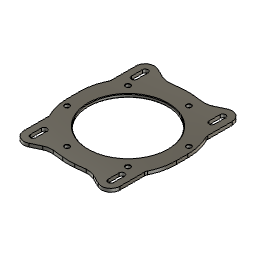
Motor_Base_Plate_Botm v4 (Autodesk Fusion 360 design; units mm, degrees)
Autodesk Fusion 360 part; units mm, degrees
sketch "Sketch1" plane through (0, 0, 0) normal (0, 0, 1) x (1, 0, 0)
  line L0 (0, 0) -> (42.0984, 0) construction
  line L1 (0, 2.5) -> (0, 20)
  line L2 (20, 0) -> (2.5, 0)
  line L3 (43.5453, 45.7571) -> (43.5453, 28.6506)
  arc A0 (32.6927, 46.2539) -> (32.6429, 45.7571) centre (35.1429, 45.7571) ccw
  arc A1 (-32.6429, 45.7571) -> (-32.7077, 46.3226) centre (-35.1429, 45.7571) ccw
  line L4 (-43.5453, 45.7571) -> (-43.5453, 28.6506)
  line L5 (16.6515, 53.2283) -> (16.6515, 59.0493) construction
  line L6 (-15.557, 53.706) -> (-15.557, 59.527) construction
  line L7 (0, 0) -> (45, 0) construction
  arc A2 (-41.8537, 25.4807) -> (-42.1265, 25.0272) centre (0, 0) ccw
  arc A3 (4.0267, 61.4469) -> (-4.7848, 61.3754) centre (-0.036, 19.1415) ccw
  arc A4 (43.4103, 49.257) -> (33.6006, 59.0168) centre (35.1429, 50.7571) ccw
  line L8 (16.6515, 58.2283) -> (16.6515, 64.0493) construction
  arc A5 (28.1023, 59.5419) -> (33.6006, 59.0168) centre (31.7651, 68.8469) ccw
  arc A6 (14.9315, 52.7652) -> (22.9245, 54.1858) centre (16.401, 67.693) ccw
  line L9 (-22.9245, 54.1858) -> (-31.3596, 58.2597)
  arc A7 (49, 5) -> (41.8537, 30.4807) centre (0, 5) ccw
  line L10 (43.5453, 50.7571) -> (43.5453, 28.6506)
  line L11 (14.9315, 52.7652) -> (5.4274, 53.7007)
  line L12 (-41.2861, 38.5638) -> (-43.4103, 49.257)
  arc A8 (-9.7818, 62.096) -> (-4.7848, 61.3754) centre (-5.9022, 71.3127) ccw
  line L13 (-14.9315, 52.7652) -> (-5.4274, 53.7007)
  arc A9 (-37.6429, 40.7571) -> (-32.6429, 40.7571) centre (-35.1429, 40.7571) ccw
  circle A10 centre (-15.557, 58.706) radius 1.5
  line L14 (-43.5453, 50.7571) -> (-43.5453, 28.6506)
  arc A11 (-44.0504, 26.4608) -> (-43.5453, 28.6506) centre (-48.5453, 28.6506) ccw
  arc A12 (-32.6429, 50.7571) -> (-37.6429, 50.7571) centre (-35.1429, 50.7571) ccw
  line L15 (-19.3563, 63.0202) -> (-28.095, 59.5544)
  arc A13 (-33.6082, 59.0182) -> (-28.095, 59.5544) centre (-31.7817, 68.85) ccw
  line L16 (-7.2407, 61.0264) -> (-0.4717, 58.2301) construction
  arc A14 (-11.79, 62.9413) -> (-19.3563, 63.0202) centre (-15.6696, 53.7246) ccw
  arc A15 (43.5453, 28.6506) -> (44.0504, 26.4608) centre (48.5453, 28.6506) ccw
  line L17 (-11.79, 62.9413) -> (-9.7818, 62.096)
  line L18 (41.2861, 38.5638) -> (43.4103, 49.257)
  arc A16 (-7.2407, 61.0264) -> (6.4194, 61.1484) centre (-0.036, 19.1415) ccw construction
  arc A17 (-22.9245, 54.1858) -> (-14.9315, 52.7652) centre (-16.401, 67.693) ccw
  arc A18 (41.2861, 38.5638) -> (41.8537, 30.4807) centre (56.0268, 35.5374) ccw
  line L19 (-15.557, 58.706) -> (-15.557, 64.527) construction
  line L20 (11.1293, 63.1457) -> (8.8867, 62.1947)
  arc A19 (4.0267, 61.4469) -> (8.8867, 62.1947) centre (4.9826, 71.4011) ccw
  line L21 (6.4194, 61.1484) -> (-0.4717, 58.2301) construction
  arc A20 (43.4103, 49.257) -> (31.3596, 58.2597) centre (35.1429, 50.7571) ccw
  line L22 (-37.6429, 50.7571) -> (-37.6429, 40.7571)
  arc A21 (-33.6006, 59.0168) -> (-43.4103, 49.257) centre (-35.1429, 50.7571) ccw
  arc A22 (-41.8537, 30.4807) -> (-41.2861, 38.5638) centre (-56.0268, 35.5374) ccw
  arc A23 (-31.3596, 58.2597) -> (-43.4103, 49.257) centre (-35.1429, 50.7571) ccw
  arc A24 (18.6963, 63.2444) -> (11.1293, 63.1457) centre (15.0335, 53.9393) ccw
  arc A25 (5.4274, 53.7007) -> (-5.4274, 53.7007) centre (0, 5) ccw
  circle A26 centre (16.6515, 58.2283) radius 1.5
  arc A27 (-41.8537, 30.4807) -> (-49, 5) centre (0, 5) ccw
  line L23 (18.6963, 63.2444) -> (28.1023, 59.5419)
  line L24 (22.9245, 54.1858) -> (31.3596, 58.2597)
  arc A28 (-33.6006, 54.0168) -> (-33.6082, 54.0182) centre (-35.1429, 45.7571) ccw
  line L25 (32.6429, 45.7571) -> (32.6429, 40.7571)
  line L26 (32.6429, 50.7571) -> (32.6429, 45.7571)
  line L27 (37.6429, 50.7571) -> (37.6429, 40.7571)
  arc A29 (37.6429, 50.7571) -> (32.6429, 50.7571) centre (35.1429, 50.7571) ccw
  arc A30 (32.6429, 40.7571) -> (37.6429, 40.7571) centre (35.1429, 40.7571) ccw
  arc A31 (-5.4274, -53.7007) -> (5.4274, -53.7007) centre (0, -5) ccw
  arc A32 (22.9245, -54.1858) -> (14.9315, -52.7652) centre (16.401, -67.693) ccw
  line L28 (-15.557, -53.706) -> (-15.557, -59.527) construction
  arc A33 (31.3596, -58.2597) -> (43.4103, -49.257) centre (35.1429, -50.7571) ccw
  line L29 (6.4194, -61.1484) -> (-0.4717, -58.2301) construction
  circle A34 centre (16.6515, -58.2283) radius 1.5
  arc A35 (-49, -5) -> (-41.8537, -30.4807) centre (0, -5) ccw
  arc A36 (-42.1265, -25.0272) -> (-41.8537, -25.4807) centre (0, 0) ccw
  line L30 (-11.79, -62.9413) -> (-9.7818, -62.096)
  arc A37 (8.8867, -62.1947) -> (4.0267, -61.4469) centre (4.9826, -71.4011) ccw
  arc A38 (-41.2861, -38.5638) -> (-41.8537, -30.4807) centre (-56.0268, -35.5374) ccw
  line L31 (11.1293, -63.1457) -> (8.8867, -62.1947)
  arc A39 (-43.5453, -28.6506) -> (-44.0504, -26.4608) centre (-48.5453, -28.6506) ccw
  line L32 (-22.9245, -54.1858) -> (-31.3596, -58.2597)
  arc A40 (-19.3563, -63.0202) -> (-11.79, -62.9413) centre (-15.6696, -53.7246) ccw
  arc A41 (-33.6082, -54.0182) -> (-33.6006, -54.0168) centre (-35.1429, -45.7571) ccw
  arc A42 (-4.7848, -61.3754) -> (4.0267, -61.4469) centre (-0.036, -19.1415) ccw
  line L33 (22.9245, -54.1858) -> (31.3596, -58.2597)
  line L34 (-15.557, -58.706) -> (-15.557, -64.527) construction
  line L35 (-43.5453, -45.7571) -> (-43.5453, -28.6506)
  line L36 (14.9315, -52.7652) -> (5.4274, -53.7007)
  arc A43 (-14.9315, -52.7652) -> (-22.9245, -54.1858) centre (-16.401, -67.693) ccw
  line L37 (43.5453, -45.7571) -> (43.5453, -28.6506)
  line L38 (-43.5453, -50.7571) -> (-43.5453, -28.6506)
  arc A44 (-43.5453, -23.6506) -> (-44.0504, -21.4608) centre (-48.5453, -23.6506) ccw
  line L39 (41.2861, -38.5638) -> (43.4103, -49.257)
  arc A45 (-28.095, -59.5544) -> (-33.6082, -59.0182) centre (-31.7817, -68.85) ccw
  arc A46 (-4.7848, -61.3754) -> (-9.7818, -62.096) centre (-5.9022, -71.3127) ccw
  line L40 (20, 0) -> (2.5, 0)
  line L41 (16.6515, -53.2283) -> (16.6515, -59.0493) construction
  line L42 (18.6963, -63.2444) -> (28.1023, -59.5419)
  arc A47 (33.6006, -59.0168) -> (43.4103, -49.257) centre (35.1429, -50.7571) ccw
  line L43 (-7.2407, -61.0264) -> (-0.4717, -58.2301) construction
  arc A48 (41.8537, -30.4807) -> (49, -5) centre (0, -5) ccw
  arc A49 (-43.4103, -49.257) -> (-33.6006, -59.0168) centre (-35.1429, -50.7571) ccw
  line L44 (16.6515, -58.2283) -> (16.6515, -64.0493) construction
  arc A50 (44.0504, -26.4608) -> (43.5453, -28.6506) centre (48.5453, -28.6506) ccw
  circle A51 centre (-15.557, -58.706) radius 1.5
  line L45 (-41.2861, -38.5638) -> (-43.4103, -49.257)
  arc A52 (41.8537, -30.4807) -> (41.2861, -38.5638) centre (56.0268, -35.5374) ccw
  arc A53 (33.6006, -59.0168) -> (28.1023, -59.5419) centre (31.7651, -68.8469) ccw
  line L46 (-19.3563, -63.0202) -> (-28.095, -59.5544)
  arc A54 (6.4194, -61.1484) -> (-7.2407, -61.0264) centre (-0.036, -19.1415) ccw construction
  line L47 (-14.9315, -52.7652) -> (-5.4274, -53.7007)
  arc A55 (-43.4103, -49.257) -> (-31.3596, -58.2597) centre (-35.1429, -50.7571) ccw
  line L48 (43.5453, -50.7571) -> (43.5453, -28.6506)
  arc A56 (11.1293, -63.1457) -> (18.6963, -63.2444) centre (15.0335, -53.9393) ccw
  line L49 (49, 5) -> (49, -5)
  line L50 (-49, -5) -> (-49, 5)
  circle A57 centre (0, 0) radius 45
  line L51 (0, 0) -> (11.6469, 43.4667) construction
  line L52 (0, 0) -> (45, 0) construction
  circle A58 centre (11.6469, 43.4667) radius 2
  circle A59 centre (-31.8198, 31.8198) radius 2
  circle A60 centre (-43.4667, -11.6469) radius 2
  circle A61 centre (-11.6469, -43.4667) radius 2
  circle A62 centre (31.8198, -31.8198) radius 2
  circle A63 centre (43.4667, 11.6469) radius 2
  circle A64 centre (0, 0) radius 35.75
  line L53 (-35.1429, 45.7571) -> (-35.1429, 50.7571)
  line L54 (-35.1429, 45.7571) -> (-35.1429, 40.7571)
  line L55 (-32.6429, 50.7571) -> (-32.6429, 40.7571)
  line L56 (37.6429, -50.7571) -> (37.6429, -40.7571)
  arc A65 (32.6429, -50.7571) -> (37.6429, -50.7571) centre (35.1429, -50.7571) ccw
  line L57 (32.6429, -50.7571) -> (32.6429, -45.7571)
  line L58 (32.6429, -45.7571) -> (32.6429, -40.7571)
  arc A66 (37.6429, -40.7571) -> (32.6429, -40.7571) centre (35.1429, -40.7571) ccw
  line L59 (-32.6429, -50.7571) -> (-32.6429, -40.7571)
  line L60 (-37.6429, -50.7571) -> (-37.6429, -40.7571)
  arc A67 (-37.6429, -50.7571) -> (-32.6429, -50.7571) centre (-35.1429, -50.7571) ccw
  line L61 (-35.1429, -45.7571) -> (-35.1429, -50.7571)
  line L62 (-35.1429, -45.7571) -> (-35.1429, -40.7571)
  arc A68 (-32.6429, -40.7571) -> (-37.6429, -40.7571) centre (-35.1429, -40.7571) ccw
  point P0 (0, 5)
  point P1 (0, 5)
  point P2 (0, -5)
  point P3 (0, -2.5)
  point P4 (0, -5)
  point P5 (42.0984, 0)
  point P6 (0, -20)
  point P7 (45, 0)
  dimension "d52" = 5.821
  dimension "d53" = 5.821
  dimension "d60" = 85
  dimension "d61" = 3
  dimension "d62" = 5.821
  dimension "d63" = 5.821
  dimension "d64" = 10
  dimension "d66" = 90
  dimension "d67" = 75
  dimension "d68" = 4
  dimension "d70" = 360
  dimension "d71" = 71.5
  constraint coincident L0.start L7.start
  constraint horizontal L0
  constraint symmetric L1 L3.start L4.start
  constraint vertical L5
  constraint vertical L6
  constraint horizontal L7
  constraint tangent L13 A17
  constraint concentric A25 A27
  constraint coincident L8.start A16
  constraint coincident A10.centre A16
  constraint coincident L8.start A26.centre
  constraint vertical L8
  constraint coincident A10.centre L19.start
  constraint vertical L19
  constraint concentric A3 A16
  constraint coincident A20.end L23
  constraint coincident A20.end A4
  constraint tangent A4 A5
  constraint tangent A5 L23
  constraint coincident L8.end L23
  constraint tangent A24 L23
  constraint tangent L20 A24
  constraint equal A5 A24
  constraint coincident A16.end L20
  constraint tangent L20 A19
  constraint tangent A3 A19
  constraint equal A5 A19
  constraint coincident L16.start L17
  constraint coincident L16.start A3
  constraint tangent A3 A8
  constraint tangent A8 L17
  constraint equal A5 A8
  constraint coincident L19.end L15
  constraint coincident L19.end L17
  constraint tangent L15 A14
  constraint tangent A14 L17
  constraint equal A5 A14
  constraint tangent L15 A13
  constraint equal A5 A13
  constraint coincident A16 A2.end
  constraint coincident A16 A1.end
  constraint coincident A16 A0.start
  constraint symmetric L1 A12.start L26.start
  constraint symmetric L1 A12.end L27.start
  constraint symmetric L1 A9.end L25.end
  constraint symmetric L1 A9.start L27.end
  constraint symmetric L1 A9 A30
  constraint symmetric L1 A12 A29
  constraint symmetric L7.start L0 A2.centre
  constraint symmetric P5 L0 L0.end
  constraint symmetric L0 L7.start A2.centre
  constraint symmetric L0 A2.start A36.end
  constraint symmetric L0 L1.start P3
  constraint symmetric L0 L1.end P6
  constraint symmetric L0 L2.start L40.start
  constraint symmetric L0 L2.end L40.end
  constraint symmetric L0 L3.start L37.start
  constraint symmetric L0 L4.start L35.start
  constraint symmetric L0 L5.start L41.start
  constraint symmetric L0 L5.end L41.end
  constraint symmetric L0 L6.start L28.start
  constraint symmetric L0 L6.end L28.end
  constraint symmetric L0 A28.end A41.start
  constraint symmetric L0 A28.start A41.end
  constraint symmetric L0 P7 L7.end
  constraint symmetric L0 A2 A36
  constraint symmetric L0 L8.end L44.end
  constraint symmetric L0 P1 P4
  constraint symmetric L0 L11.end A31.end
  constraint symmetric L0 L12.start A38.start
  constraint symmetric L0 A15.end A50.start
  constraint symmetric L0 A4.end A47.start
  constraint symmetric L0 A4.start A33.end
  constraint symmetric L0 L8.start A34.centre
  constraint symmetric L0 L20.start L31.start
  constraint symmetric L0 A16.end L29.start
  constraint symmetric L0 L18.start L39.start
  constraint symmetric L0 A20.end A33.start
  constraint symmetric L0 A7.end A48.start
  constraint symmetric L0 A3.start A37.end
  constraint symmetric L0 L20.end A37.start
  constraint symmetric L0 A6.end A32.start
  constraint symmetric L0 L9.start L32.start
  constraint symmetric L0 A24.start L42.start
  constraint symmetric L0 L14.start L38.start
  constraint symmetric L0 A3.end A42.start
  constraint symmetric L0 L9.end L32.end
  constraint symmetric L0 L4.end A39.start
  constraint symmetric L0 L12.end A49.start
  constraint symmetric L0 A7.start A48.end
  constraint symmetric L0 A5.start L42.end
  constraint symmetric L0 A11.start A39.end
  constraint symmetric L0 L13.end A31.start
  constraint symmetric L0 L16.start L43.start
  constraint symmetric L0 A21.start A49.end
  constraint symmetric L0 L19.end L34.end
  constraint symmetric L0 A10.centre L34.start
  constraint symmetric L0 L3.end L37.end
  constraint symmetric L0 L15.start A40.start
  constraint symmetric L0 A8.start L30.end
  constraint symmetric L0 A14.start L30.start
  constraint symmetric L0 A22.start A35.end
  constraint symmetric L0 A6.start A32.end
  constraint symmetric L0 L15.end A45.start
  constraint symmetric L0 L10.start L48.start
  constraint symmetric L0 A27.end A35.start
  constraint symmetric L0 L13.start A43.start
  constraint symmetric L0 L16.end L29.end
  constraint symmetric L0 A13.start A45.end
  constraint symmetric L0 A3 A42
  constraint symmetric L0 A4 A47
  constraint symmetric L0 A5 A53
  constraint symmetric L0 A6 A32
  constraint symmetric L0 A7 A48
  constraint symmetric L0 A8 A46
  constraint symmetric L0 A10 A51
  constraint symmetric L0 A11 A39
  constraint symmetric L0 A13 A45
  constraint symmetric L0 A14 A40
  constraint symmetric L0 A15 A50
  constraint symmetric L0 A16 A54
  constraint symmetric L0 A17 A43
  constraint symmetric L0 A18 A52
  constraint symmetric L0 A19 A37
  constraint symmetric L0 A20 A33
  constraint symmetric L0 A21 A49
  constraint symmetric L0 A22 A38
  constraint symmetric L0 A23 A55
  constraint symmetric L0 A24 A56
  constraint symmetric L0 A25 A31
  constraint symmetric L0 A26 A34
  constraint symmetric L0 A27 A35
  constraint symmetric L0 A2.end A36.start
  constraint symmetric L0 A28 A41
  constraint tangent A48 L49
  constraint tangent A27 L50
  constraint horizontal L52
  constraint coincident L51.end A58.centre
  constraint concentric A2 A64
  constraint coincident A1.centre A28.centre
  constraint coincident A12.centre A21.centre
  constraint coincident A9.centre L54.end
  constraint parallel L53 L54
  constraint symmetric A12.end L53 A12.start
  constraint symmetric A9.start L53 A9.end
  constraint symmetric A12.start L40 L59.start
  constraint symmetric A12.end L40 L60.start
  constraint symmetric A9.end L40 L59.end
  constraint symmetric A9.start L40 L60.end
  constraint symmetric A9 L40 A68
  constraint symmetric A12 L40 A67
  constraint symmetric A0.end L40 L57.end
  constraint symmetric L25.end L40 L58.end
  constraint symmetric L26.start L40 A65.start
  constraint symmetric L27.start L40 L56.start
  constraint symmetric L27.end L40 L56.end
  constraint symmetric A29 L40 A65
  constraint symmetric A30 L40 A66
  constraint symmetric L40 A1.centre A41.centre
  constraint symmetric L40 A12.centre A49.centre
  constraint symmetric L40 A9.centre L62.end
  constraint symmetric L40 A12.start L59.start
  constraint symmetric L40 A9.end L59.end
  measures "d52" distance of L5.start L5.end
  measures "d53" distance of L6.start L6.end
  measures "d60" diameter of A16
  measures "d61" diameter of A26
  measures "d62" distance of L8.end L8.start
  measures "d63" distance of L19.end A10.centre
  measures "d64" radius of A5
  measures "d66" diameter of A57
  measures "d67" angle of L51 L52
  measures "d68" diameter of A58
  measures "d71" diameter of A64
extrude "Extrude1" add sketch "Sketch1" along normal blind 3 contours L3 A4 A7 L10 A15 L18 A18 A20 | A4 A6 L9 A7 L11 L12 L13 A13 L18 A17 A18 A20 A21 A22 A23 A25 A27 L24 A31 A32 A33 A35 A38 L32 L33 L36 A43 L39 A45 A47 A48 A49 L45 A52 L47 A55 L49 L50 | A33 L37 L39 A47 A48 A50 A52 L48 | L4 L12 L14 A11 A21 A22 A23 A27 | A35 A38 A39 L35 L38 A49 L45 A55 | A57 A58 A59 A60 A61 A62 A63
chamfer "Chamfer1" distance 0.25 angle 45 12 edges at (-13.5115, -42.7434, 0) (-13.5115, -42.7434, 3) (-45.3313, -10.9236, 0) (-45.3313, -10.9236, 3) (-33.6845, 32.543, 0) (-33.6845, 32.543, 3) (9.7822, 44.1899, 3) (9.7822, 44.1899, 0) (41.602, 12.3701, 0) (29.9552, -31.0966, 0) (29.9552, -31.0966, 3) (41.602, 12.3701, 3)
chamfer "Chamfer1" distance 0.5 angle 45 1 faces at (-35.5724, -3.5596, 1)
thread "Thread3" [suppressed]
equation "d67 = 90 deg - 15 deg"
